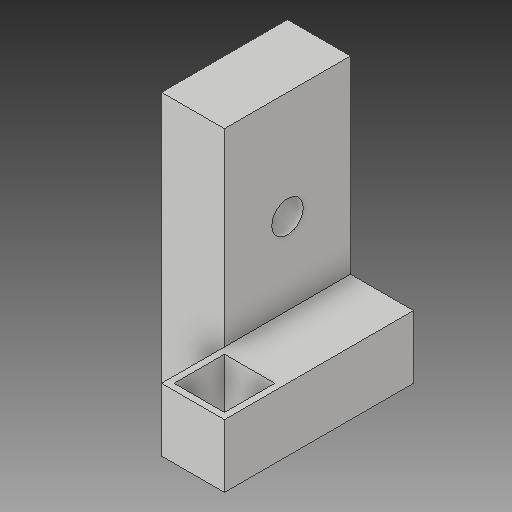
# Autodesk Inventor part: intakee mount
Saved by Autodesk Inventor 2017 (Build 210142000, 142)
## iProperties
Created: 2020-02-01
Part Number: intakee mount
Material: Generic
Document SubType Name: Modeling
Designer: S346553810
Density: 1 g/cm^3
Appearance: Default
Author: S346553810
Autodesk Inventor part; units mm, degrees
ref_plane "YZ Plane" through (0, 0, 0) normal (1, 0, 0) x (0, 1, 0)
ref_plane "XZ Plane" through (0, 0, 0) normal (0, 1, 0) x (-1, 0, 0)
ref_plane "XY Plane" through (0, 0, 0) normal (0, 0, 1) x (1, 0, 0)
sketch "Sketch1" plane through (0, 0, 0) normal (0, 1, 0) x (-1, 0, 0)
  line L0 (25.4, 231.775) -> (25.4, 257.175)
  line L1 (25.4, 257.175) -> (0, 257.175)
  line L2 (0, 231.775) -> (0, 257.175)
  line L3 (25.4, 231.775) -> (0, 231.775)
  line L4 (2.54, 234.315) -> (2.54, 254.635)
  line L5 (2.54, 254.635) -> (22.86, 254.635)
  line L6 (22.86, 254.635) -> (22.86, 234.315)
  line L7 (22.86, 234.315) -> (2.54, 234.315)
  line L8 (25.4, 231.775) -> (0, 231.775)
  line L9 (0, 231.775) -> (0, 180.975)
  line L10 (0, 180.975) -> (25.4, 180.975)
  line L11 (25.4, 180.975) -> (25.4, 231.775)
  line L12 (25.4, 231.775) -> (25.4, 257.175)
  line L13 (25.4, 257.175) -> (0, 257.175)
  line L14 (0, 231.775) -> (0, 257.175)
  line L15 (25.4, 231.775) -> (0, 231.775)
  line L16 (2.54, 234.315) -> (2.54, 254.635)
  line L17 (2.54, 254.635) -> (22.86, 254.635)
  line L18 (22.86, 254.635) -> (22.86, 234.315)
  line L19 (22.86, 234.315) -> (2.54, 234.315)
  line L20 (25.4, 231.775) -> (0, 231.775)
  line L21 (0, 231.775) -> (0, 180.975)
  line L22 (0, 180.975) -> (25.4, 180.975)
  line L23 (25.4, 180.975) -> (25.4, 231.775)
  point P0 (0, 0)
  dimension "d0" = 50.8
  dimension "d1" = 50.8
  constraints: 16 end point, 4 parallel, 2 horizontal, 2 perpendicular
  measures "d0" distance of L9.end L8.end
  measures "d1" distance of L21.end L20.end
extrude "Extrusion1" add sketch "Sketch1" along normal blind 25.4
sketch "Sketch2" plane through (0, 0, 0) normal (0, -1, 0) x (1, 0, 0)
  line L0 (-25.4, 180.975) -> (-25.4, 257.175) projected
  line L1 (-25.4, 180.975) -> (-50.8, 180.975)
  line L2 (-50.8, 180.975) -> (-50.8, 231.775)
  line L3 (-50.8, 231.775) -> (-25.4, 231.775)
  line L4 (-25.4, 231.775) -> (-25.4, 180.975)
  point P0 (0, 0)
  dimension "d4" = 25.4
  dimension "d5" = 50.8
  constraints: 8 end point, 2 parallel, 1 horizontal, 1 perpendicular
  measures "d4" distance of L2.end L3.end
  measures "d5" distance of L1.end L2.end
extrude "Extrusion2" add sketch "Sketch2" against normal blind 101.6
sketch "Sketch5" plane through (-50.8, 0, 180.975) normal (-1, 0, 0) x (0, 0, 1)
  circle A0 centre (25.4, 19.05) radius 6.35 construction
  line L0 (25.4, 19.05) -> (25.4, 58.166) construction
  circle A1 centre (25.4, 58.166) radius 6.35
  point P0 (-180.975, 0)
  dimension "d10" = 39.116
  dimension "d11" = 12.7
  constraints: 2 centre point, 2 end point, 1 coincident, 1 vertical, 2 other
  measures "d10" distance of L0.start L0.end
  measures "d11" diameter of A1
extrude "Extrusion4" cut sketch "Sketch5" against normal blind 25.4
body "Solid1"
